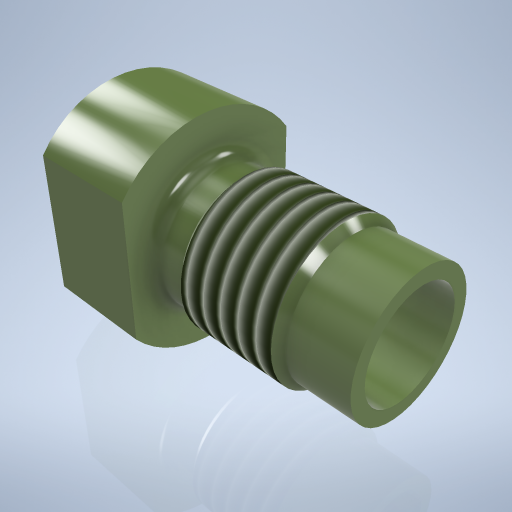
# Autodesk Inventor part: Arbeitszylinder
Saved by Autodesk Inventor 2024.2 (Build 282272000, 272)
## iProperties
Created: 2024-04-22
Part Number: Arbeitszylinder
Material: Titan
Document SubType Name: Modeling
Designer: Fabri
Density: 4.51 g/cm^3
Appearance: Dunkeloliv
Author: Fabri
Autodesk Inventor part; units mm, degrees
ref_plane "YZ Plane" through (0, 0, 0) normal (1, 0, 0) x (0, 1, 0)
ref_plane "XZ Plane" through (0, 0, 0) normal (0, 1, 0) x (-1, 0, 0)
ref_plane "XY Plane" through (0, 0, 0) normal (0, 0, 1) x (1, 0, 0)
sketch "Skizze1" plane through (0, 0, 0) normal (0, 0, 1) x (1, 0, 0)
  line L0 (0, 0) -> (42, 0)
  line L1 (0, 0) -> (0, 15)
  line L2 (0, 15) -> (14, 15)
  line L3 (14, 15) -> (14, 9)
  line L4 (14, 9) -> (19, 9)
  line L5 (19, 9) -> (20, 10)
  line L6 (20, 10) -> (33, 10)
  line L7 (33, 10) -> (34, 9)
  line L8 (34, 9) -> (42, 9)
  line L9 (42, 9) -> (42, 0)
  dimension "d0" = 45
  dimension "d1" = 42
  dimension "d2" = 20
  dimension "d3" = 18
  dimension "d4" = 5
  dimension "d5" = 28
  dimension "d6" = 8
  dimension "d7" = 30
  constraints: 20 end point, 5 perpendicular, 2 horizontal, 1 horizontal alignment, 1 parallel, 1 vertical
  measures "d0" angle of L7 L8
  measures "d1" distance of L0.start L0.end
  measures "d2" diameter of L6.end L0
  measures "d3" diameter of L8 L0
  measures "d4" distance of L4.end L3.end
  measures "d5" distance between parallel lines of L9 L3
  measures "d6" distance of L7.end L8.end
  measures "d7" diameter of L2 L0
revolve "Umdrehung1" add sketch "Skizze1" angle 360 about axis through (0, 0, 0) along (1, 0, 0)
thread "Gewinde1" size "M20x2.5" class "6g" standard "ISO Metric profile" full length
sketch "Skizze2" plane through (0, 0, 0) normal (-1, 0, 0) x (0, 0, 1)
  circle A0 centre (0, 0) radius 15 projected
  constraints: 1 coincident
hole "Bohrung1" at (0, 0, 0) direction (1, 0, 0) diameter 14 depth 42
sketch "Skizze3" plane through (0, 0, 0) normal (-1, 0, 0) x (0, 0, 1)
  circle A0 centre (0, 0) radius 15 projected
  line L0 (9, 12) -> (-9, 12)
  circle A1 centre (0, 0) radius 15 projected
  line L1 (9, -12) -> (-9, -12)
  line L2 (15, 0) -> (-15, 0) construction
  point P0 (-9, -12)
  point P1 (-9, 12)
  dimension "d18" = 24
  constraints: 6 end point, 5 point on circle, 2 parallel, 1 horizontal, 1 midpoint, 3 other
  measures "d18" distance between parallel lines of L1 L0
extrude "Extrusion1" cut sketch "Skizze3" against normal up to surface (14 mm away) contours L0 A0 | A0 L1
fillet "Rundung1" radius 2 1 edges at (14, -9, 0)
